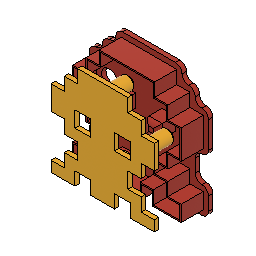
8bit Alien Cutter v6 (Autodesk Fusion 360 design; units mm, degrees)
Autodesk Fusion 360 part; units mm, degrees
sketch "Sketch1" plane through (0, 0, 0) normal (0, 0, 1) x (1, 0, 0)
  line L0 (-6, 0) -> (-6, 6)
  line L1 (-6, 6) -> (-12, 6)
  line L2 (-12, 6) -> (-12, 0)
  line L3 (-12, 0) -> (-24, 0)
  line L4 (-24, 0) -> (-24, 6)
  line L5 (-24, 6) -> (-18, 6)
  line L6 (-18, 6) -> (-18, 12)
  line L7 (-18, 12) -> (-12, 12)
  line L8 (-12, 12) -> (-12, 18)
  line L9 (-12, 18) -> (-18, 18)
  line L10 (-18, 18) -> (-18, 24)
  line L11 (-18, 24) -> (-24, 24)
  line L12 (-24, 24) -> (-24, 36)
  line L13 (-24, 36) -> (-18, 36)
  line L14 (-18, 36) -> (-18, 42)
  line L15 (-18, 42) -> (-12, 42)
  line L16 (-12, 42) -> (-12, 48)
  line L17 (-12, 48) -> (0, 48)
  line L18 (0, 48) -> (0, 0) construction
  line L19 (0, 0) -> (-6, 0)
  line L20 (-12, 24) -> (-6, 24)
  line L21 (-6, 24) -> (-6, 30)
  line L22 (-6, 30) -> (-12, 30)
  line L23 (-12, 30) -> (-12, 24)
  line L24 (0, -3) -> (-9, -3)
  line L25 (-9, -3) -> (-27, -3)
  line L26 (-27, -3) -> (-27, 9)
  line L27 (-27, 9) -> (-21, 9)
  line L28 (-21, 9) -> (-21, 15)
  line L29 (-21, 15) -> (-21, 21)
  line L30 (-21, 21) -> (-27, 21)
  line L31 (-27, 21) -> (-27, 39)
  line L32 (-27, 39) -> (-21, 39)
  line L33 (-21, 39) -> (-21, 45)
  line L34 (-21, 45) -> (-15, 45)
  line L35 (-15, 45) -> (-15, 51)
  line L36 (-15, 51) -> (0, 51)
  line L37 (0, -0.6) -> (-6.6, -0.6)
  line L38 (-6.6, -0.6) -> (-6.6, 5.4)
  line L39 (-6.6, 5.4) -> (-11.4, 5.4)
  line L40 (-11.4, 5.4) -> (-11.4, -0.6)
  line L41 (-11.4, -0.6) -> (-24.6, -0.6)
  line L42 (-24.6, -0.6) -> (-24.6, 6.6)
  line L43 (-24.6, 6.6) -> (-18.6, 6.6)
  line L44 (-18.6, 6.6) -> (-18.6, 12.6)
  line L45 (-18.6, 12.6) -> (-12.6, 12.6)
  line L46 (-12.6, 12.6) -> (-12.6, 17.4)
  line L47 (-12.6, 17.4) -> (-18.6, 17.4)
  line L48 (-18.6, 17.4) -> (-18.6, 23.4)
  line L49 (-18.6, 23.4) -> (-24.6, 23.4)
  line L50 (-24.6, 23.4) -> (-24.6, 36.6)
  line L51 (-24.6, 36.6) -> (-18.6, 36.6)
  line L52 (-18.6, 36.6) -> (-18.6, 42.6)
  line L53 (-18.6, 42.6) -> (-12.6, 42.6)
  line L54 (-12.6, 42.6) -> (-12.6, 48.6)
  line L55 (-12.6, 48.6) -> (0, 48.6)
  line L56 (0, 0.6) -> (-5.4, 0.6)
  line L57 (-5.4, 0.6) -> (-5.4, 6.6)
  line L58 (-5.4, 6.6) -> (-12.6, 6.6)
  line L59 (-12.6, 6.6) -> (-12.6, 0.6)
  line L60 (-12.6, 0.6) -> (-23.4, 0.6)
  line L61 (-23.4, 0.6) -> (-23.4, 5.4)
  line L62 (-23.4, 5.4) -> (-17.4, 5.4)
  line L63 (-17.4, 5.4) -> (-17.4, 11.4)
  line L64 (-17.4, 11.4) -> (-11.4, 11.4)
  line L65 (-11.4, 11.4) -> (-11.4, 18.6)
  line L66 (-11.4, 18.6) -> (-17.4, 18.6)
  line L67 (-17.4, 18.6) -> (-17.4, 24.6)
  line L68 (-17.4, 24.6) -> (-23.4, 24.6)
  line L69 (-23.4, 24.6) -> (-23.4, 35.4)
  line L70 (-23.4, 35.4) -> (-17.4, 35.4)
  line L71 (-17.4, 35.4) -> (-17.4, 41.4)
  line L72 (-17.4, 41.4) -> (-11.4, 41.4)
  line L73 (-11.4, 41.4) -> (-11.4, 47.4)
  line L74 (-11.4, 47.4) -> (0, 47.4)
  line L75 (0, 51) -> (0, -3)
  circle A0 centre (-18, 30) radius 3
  circle A1 centre (0, 42) radius 3
  circle A2 centre (0, 12) radius 3
  circle A3 centre (-18, 30) radius 3.5
  circle A4 centre (0, 42) radius 3.5
  circle A5 centre (0, 12) radius 3.5
  line L76 (-12.6, 23.4) -> (-5.4, 23.4)
  line L77 (-5.4, 23.4) -> (-5.4, 30.6)
  line L78 (-5.4, 30.6) -> (-12.6, 30.6)
  line L79 (-12.6, 30.6) -> (-12.6, 23.4)
  dimension "d1" = 6
  dimension "d2" = 12
  dimension "d3" = 12
  dimension "d4" = 12
  dimension "d5" = 6
  dimension "d8" = -3
  dimension "d9" = -0.6
  dimension "d10" = 0.6
  dimension "d11" = 6
  dimension "d18" = 7
  dimension "d25" = 0.6
  constraint vertical L0
  constraint perpendicular L0 L1
  constraint perpendicular L1 L2
  constraint perpendicular L2 L3
  constraint perpendicular L3 L4
  constraint perpendicular L4 L5
  constraint perpendicular L5 L6
  constraint perpendicular L4 L7
  constraint perpendicular L7 L8
  constraint perpendicular L8 L9
  constraint perpendicular L9 L10
  constraint perpendicular L8 L11
  constraint perpendicular L11 L12
  constraint perpendicular L12 L13
  constraint perpendicular L13 L14
  constraint perpendicular L12 L15
  constraint perpendicular L15 L16
  constraint perpendicular L12 L17
  constraint coincident L18.end L19.start
  constraint perpendicular L17 L18
  constraint perpendicular L0 L19
  constraint perpendicular L0 L20
  constraint perpendicular L20 L21
  constraint perpendicular L21 L22
  constraint perpendicular L20 L23
  constraint equal L0 L19
  constraint equal L0 L1
  constraint equal L1 L2
  constraint equal L2 L4
  constraint equal L4 L5
  constraint equal L6 L7
  constraint equal L7 L8
  constraint equal L8 L9
  constraint equal L9 L10
  constraint equal L10 L11
  constraint equal L11 L13
  constraint equal L13 L14
  constraint equal L14 L15
  constraint equal L15 L16
  constraint equal L22 L23
  constraint collinear L11 L20
  constraint collinear L0 L21
  constraint perpendicular L55 L75
  constraint equal A0 A1
  constraint equal A1 A2
  constraint vertical L13.end A0.centre
  constraint horizontal L22.end A0.centre
  constraint vertical A1.centre A2.centre
  constraint vertical L18.end A2.centre
  constraint horizontal L7.end A2.centre
  constraint horizontal L15.end A1.centre
  constraint concentric A0 A3
  constraint concentric A1 A4
  constraint concentric A2 A5
  constraint equal A3 A4
  constraint equal A3 A5
  measures "d1" distance of L0.start L18.end
  measures "d2" distance of L2.end L3.end
  measures "d3" distance of L11.end L12.end
  measures "d4" distance of L16.end L17.end
  measures "d5" distance of L21.end L22.end
  measures "d11" diameter of A0
  measures "d18" diameter of A3
extrude "Extrude1" add sketch "Sketch1" against normal blind 2 contours L0 L1 L2 L3 L4 L5 L6 L7 L8 L9 L10 L11 L12 L13 L14 L15 L16 L17 L19 L37 L38 L39 L40 L41 L42 L43 L44 L45 L46 L47 L48 L49 L50 L51 L52 L53 L54 L55 L75 | L0 L1 L2 L3 L4 L5 L6 L7 L8 L9 L10 L11 L12 L13 L14 L15 L16 L17 L19 L56 L57 L58 L59 L60 L61 L62 L63 L64 L65 L66 L67 L68 L69 L70 L71 L72 L73 L74 L75 | L56 L57 L58 L59 L60 L61 L62 L63 L64 L65 L66 L67 L68 L69 L70 L71 L72 L73 L74 L75 A4 A5 | L24 L25 L26 L27 L28 L29 L30 L31 L32 L33 L34 L35 L36 L37 L38 L39 L40 L41 L42 L43 L44 L45 L46 L47 L48 L49 L50 L51 L52 L53 L54 L55 L75 | L20 L21 L22 L23 | L76 L77 L78 L79 makes body 1
extrude "Extrude2" add sketch "Sketch1" along normal blind 10 contours L0 L1 L2 L3 L4 L5 L6 L7 L8 L9 L10 L11 L12 L13 L14 L15 L16 L17 L19 L37 L38 L39 L40 L41 L42 L43 L44 L45 L46 L47 L48 L49 L50 L51 L52 L53 L54 L55 L75 bodies 1
extrude "Extrude3" add sketch "Sketch1" along normal blind 8 contours L20 L21 L22 L23 bodies 1
fillet "Fillet1" radius 3 10 edges at (-27, 39, -1) (-21, 39, -1) (-21, 45, -1) (-15, 45, -1) (-15, 51, -1) (-27, 21, -1) (-21, 21, -1) (-21, 9, -1) (-27, 9, -1) (-27, -3, -1) on bodies 1
fillet "Fillet2" radius 2 1 faces at (-10, 26, 8) on bodies 1
mirror "Mirror1" about plane through (0, 0, 0) normal (1, 0, 0) of bodies 1 merged
extrude "Extrude1'" add sketch "Sketch1" along normal blind 2 separate body contours L56 L57 L58 L59 L60 L61 L62 L63 L64 L65 L66 L67 L68 L69 L70 L71 L72 L73 L74 L75 A4 A5 | L75 A2 A5 | L75 A2 | L75 A1 A4 | L75 A1 | A0 | A3 picked at (-0.3229, 8.6909) picked at (-0.7818, 11.3765) picked at (-0.8125, 45.224) picked at (-2.0575, 41.6347) makes body 2 in component "Ejector"
extrude "Extrude2'" add sketch "Sketch1" against normal blind 10 contours L75 A2 | L75 A1 | A0 picked at (-0.7818, 11.3765) picked at (-2.0575, 41.6347) bodies 2 in component "Ejector"
mirror "Mirror1'" about plane through (0, 0, 0) normal (1, 0, 0) of bodies 2 merged in component "Ejector"
chamfer "Chamfer1" distance 1 angle 45 4 edges at (20.797, 31.0848, -10) (-2.797, 43.0848, -10) (2.797, 13.0848, -10) (-20.797, 31.0848, -10) on bodies 2 in component "Ejector"
component "Ejector" placed x (1, 0, 0) y (0, 1, 0) z (0, 0, 1) at (0, 0, 18.984)
equation "d1 = modul"
equation "d2 = 2 * d1"
equation "d3 = d2"
equation "d4 = d3"
equation "d5 = d1"
equation "modul = 6 mm"
equation "radius = 2 mm"
named bodies: "Form", "Ejector"
